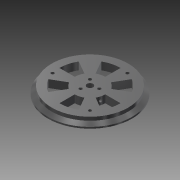
# Autodesk Inventor part: wheel small
Saved by Autodesk Inventor 2011 (Build 150239000, 239)
## iProperties
Created: 2010-04-18
Part Number: wheel small
Document SubType Name: Modeling
Designer: lucio
Density: 0.94 g/cm^3
Material: UHMW, Black
Mass: 59.969 g
Surface Area: 231.254 cm^2
Volume: 63.7969 cm^3
GlobalPropertyList: <PropertyList/>
Author: lucio
Autodesk Inventor part; units mm, degrees
ref_plane "YZ Plane" through (0, 0, 0) normal (1, 0, 0) x (0, 1, 0)
ref_plane "XZ Plane" through (0, 0, 0) normal (0, 1, 0) x (-1, 0, 0)
sketch "Sketch1" plane through (0, 0, 0) normal (0, 0, 1) x (1, 0, 0)
  circle A0 centre (0, 0) radius 55
  circle A1 centre (0, 0) radius 50
  circle A2 centre (0, 0) radius 4
  line L0 (0, 20) -> (0, 40)
  arc A3 (0, 20) -> (-10, 17.3205) centre (0, 0) ccw
  line L1 (0, 0) -> (-10, 17.3205) construction
  line L2 (0, 0) -> (0, 20) construction
  arc A4 (0, 40) -> (-20, 34.641) centre (0, 0) ccw
  line L3 (0, 0) -> (-20, 34.641) construction
  line L4 (0, 0) -> (0, 40) construction
  line L5 (-10, 17.3205) -> (-20, 34.641)
  line L6 (-17.3205, 10) -> (-34.641, 20)
  arc A5 (-17.3205, 10) -> (-20, 0) centre (0, 0) ccw
  line L7 (0, 0) -> (-20, 0) construction
  line L8 (0, 0) -> (-17.3205, 10) construction
  arc A6 (-34.641, 20) -> (-40, 0) centre (0, 0) ccw
  line L9 (0, 0) -> (-40, 0) construction
  line L10 (0, 0) -> (-34.641, 20) construction
  line L11 (-20, 0) -> (-40, 0)
  line L12 (-17.3205, -10) -> (-34.641, -20)
  arc A7 (-17.3205, -10) -> (-10, -17.3205) centre (0, 0) ccw
  line L13 (0, 0) -> (-10, -17.3205) construction
  line L14 (0, 0) -> (-17.3205, -10) construction
  arc A8 (-34.641, -20) -> (-20, -34.641) centre (0, 0) ccw
  line L15 (0, 0) -> (-20, -34.641) construction
  line L16 (0, 0) -> (-34.641, -20) construction
  line L17 (-10, -17.3205) -> (-20, -34.641)
  line L18 (0, -20) -> (0, -40)
  arc A9 (0, -20) -> (10, -17.3205) centre (0, 0) ccw
  line L19 (0, 0) -> (10, -17.3205) construction
  line L20 (0, 0) -> (0, -20) construction
  arc A10 (0, -40) -> (20, -34.641) centre (0, 0) ccw
  line L21 (0, 0) -> (20, -34.641) construction
  line L22 (0, 0) -> (0, -40) construction
  line L23 (10, -17.3205) -> (20, -34.641)
  line L24 (17.3205, -10) -> (34.641, -20)
  arc A11 (17.3205, -10) -> (20, 0) centre (0, 0) ccw
  line L25 (0, 0) -> (20, 0) construction
  line L26 (0, 0) -> (17.3205, -10) construction
  arc A12 (34.641, -20) -> (40, 0) centre (0, 0) ccw
  line L27 (0, 0) -> (40, 0) construction
  line L28 (0, 0) -> (34.641, -20) construction
  line L29 (20, 0) -> (40, 0)
  line L30 (17.3205, 10) -> (34.641, 20)
  arc A13 (17.3205, 10) -> (10, 17.3205) centre (0, 0) ccw
  line L31 (0, 0) -> (10, 17.3205) construction
  line L32 (0, 0) -> (17.3205, 10) construction
  arc A14 (34.641, 20) -> (20, 34.641) centre (0, 0) ccw
  line L33 (0, 0) -> (20, 34.641) construction
  line L34 (0, 0) -> (34.641, 20) construction
  line L35 (10, 17.3205) -> (20, 34.641)
  point P0 (0, 10)
  point P1 (-2.5882, 9.6593)
  point P2 (-5, 8.6603)
  point P3 (-7.0711, 7.0711)
  point P4 (-8.6603, 5)
  point P5 (-9.6593, 2.5882)
  point P6 (-10, 0)
  point P7 (-9.6593, -2.5882)
  point P8 (-8.6603, -5)
  point P9 (-7.0711, -7.0711)
  point P10 (-5, -8.6603)
  point P11 (-2.5882, -9.6593)
  point P12 (0, -10)
  point P13 (2.5882, -9.6593)
  point P14 (5, -8.6603)
  point P15 (7.0711, -7.0711)
  point P16 (8.6603, -5)
  point P17 (9.6593, -2.5882)
  point P18 (10, 0)
  point P19 (9.6593, 2.5882)
  point P20 (8.6603, 5)
  point P21 (7.0711, 7.0711)
  point P22 (5, 8.6603)
  point P23 (2.5882, 9.6593)
  point P24 (10.3528, -38.637)
  point P25 (20, -34.641)
  point P26 (28.2843, -28.2843)
  point P27 (34.641, -20)
  point P28 (38.637, -10.3528)
  point P29 (40, 0)
  point P30 (38.637, 10.3528)
  point P31 (34.641, 20)
  point P32 (28.2843, 28.2843)
  point P33 (20, 34.641)
  point P34 (10.3528, 38.637)
  point P35 (0, 40)
  point P36 (-10.3528, 38.637)
  point P37 (-20, 34.641)
  point P38 (-28.2843, 28.2843)
  point P39 (-34.641, 20)
  point P40 (-38.637, 10.3528)
  point P41 (-40, 0)
  point P42 (-38.637, -10.3528)
  point P43 (-34.641, -20)
  point P44 (-28.2843, -28.2843)
  point P45 (-20, -34.641)
  point P46 (-10.3528, -38.637)
  dimension "d1" = 100
  dimension "d2" = 8
  dimension "d11" = 20
  dimension "d12" = 20
  dimension "d13" = 30
  dimension "d14" = 30
  dimension "d17" = 360
  dimension "d34" = 10
  dimension "d37" = 360
  dimension "d48" = 360
  dimension "d57" = 110
  constraints: 72 end point, 24 point on circle, 15 centre point, 13 coincident, 1 collinear, 1 point on line, 1 vertical, 133 other
  measures "d1" diameter of A1
  measures "d2" diameter of A2
  measures "d11" distance of L0.start L0.end
  measures "d12" distance of point (0, 0) L0.start
  measures "d13" angle of L2 L1
  measures "d14" angle of L4 L3
  measures "d34" distance of point (0, 0) point (0, 10)
  measures "d57" diameter of A0
extrude "Extrusion1" add sketch "Sketch1" along normal blind 10 contours A1
extrude "Extrusion2" add sketch "Sketch1" along normal blind 5.5 contours A0
hole "Hole2" at (-2.5882, -9.6593, 0) at (-7.0711, 7.0711, 0) at (9.6593, 2.5882, 0) direction (0, 0, 1) diameter 4 end through all counterbore diameter 7 counterbore depth 4
hole "Hole3" at (28.2843, -28.2843, 0) at (-38.637, -10.3528, 0) at (10.3528, 38.637, 0) direction (0, 0, 1) diameter 4 end through all counterbore diameter 7 counterbore depth 4
chamfer "Chamfer2" distance 3.5 distance2 5 1 edges at (-55, 0, 5.5) measured on face at (-50.386, -22.0512, 3.6667)
ref_plane "Work Plane3" through (19.3185, -5.1764, 0) normal (-0.9659, 0.2588, 0) x (-0.2588, -0.9659, 0)
sketch "Sketch3" plane through (19.3185, -5.1764, 0) normal (-0.9659, 0.2588, 0) x (-0.2588, -0.9659, 0)
  point P0 (0, 0)
  point P1 (0, 5)
  dimension "d61" = 5
  measures "d61" distance of point (0, 0) point (0, 5)
hole "Hole4" at (19.3185, -5.1764, 5) direction (-0.9659, 0.2588, 0) diameter 3.5 depth 20
body "Solid1"
